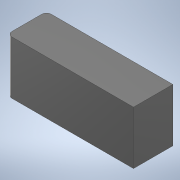
# Autodesk Inventor part: turnigy_graphene_12Ah
Saved by Autodesk Inventor 2020.2 (Build 242310000, 310)
## iProperties
Created: 2020-08-25
Part Number: turnigy_graphene_12Ah
Material: Generic
Document SubType Name: Modeling
Designer: Krishna Makhija
Density: 1 g/cm^3
Appearance: Default
Author: Krishna Makhija
Autodesk Inventor part; units mm, degrees
ref_plane "YZ Plane" through (0, 0, 0) normal (1, 0, 0) x (0, 1, 0)
ref_plane "XZ Plane" through (0, 0, 0) normal (0, 1, 0) x (-1, 0, 0)
ref_plane "XY Plane" through (0, 0, 0) normal (0, 0, 1) x (1, 0, 0)
sketch "Sketch1" plane through (0, 0, 0) normal (0, 0, 1) x (1, 0, 0)
  point P0 (0, 0)
sketch "Sketch2" plane through (0, 0, 0) normal (0, 0, 1) x (1, 0, 0)
  line L0 (-91.5002, 38.5) -> (91.5002, 38.5)
  line L1 (91.5002, 38.5) -> (91.5002, -38.5)
  line L2 (91.5002, -38.5) -> (-91.5002, -38.5)
  line L3 (-91.5002, -38.5) -> (-91.5002, 38.5)
  line L4 (-91.5002, 38.5) -> (91.5002, -38.5) construction
  line L5 (91.5002, 38.5) -> (-91.5002, -38.5) construction
  point P0 (0, 0)
  constraints: 12 end point, 2 midpoint, 2 parallel, 1 horizontal, 1 perpendicular
extrude "Extrusion1" add sketch "Sketch2" along normal blind 57
fillet "Fillet1" radius 7 2 edges at (-91.5002, 0, 57) (-91.5002, 0, 0)
body "Solid1"
